Autodesk Fusion 360 part; units mm, degrees
(part 3 of 5)
  spline S763 degree 3 poles (27.3731, 3.8659) (27.3731, 3.7395) (27.3641, 3.6132) (27.346, 3.5681) knots 0 0 0 0 1 1 1 1
  spline S764 degree 3 poles (27.346, 3.5681) (27.337, 3.532) (26.967, 3.4959) (26.5157, 3.4868) knots 0 0 0 0 1 1 1 1
  spline S765 degree 3 poles (26.5157, 3.4868) (26.0645, 3.4778) (25.6222, 3.4598) (25.532, 3.4598) knots 0 0 0 0 1 1 1 1
  spline S766 degree 3 poles (25.532, 3.4598) (25.4327, 3.4507) (25.1981, 3.6132) (24.9995, 3.8208) knots 0 0 0 0 1 1 1 1
  spline S767 degree 3 poles (24.9995, 3.8208) (24.6566, 4.1727) (24.4851, 4.263) (24.4851, 4.1005) knots 0 0 0 0 1 1 1 1
  spline S768 degree 3 poles (24.4851, 4.1005) (24.4851, 4.0554) (24.5483, 3.9742) (24.6205, 3.911) knots 0 0 0 0 1 1 1 1
  spline S769 degree 3 poles (24.6205, 3.911) (24.9183, 3.6673) (24.7288, 3.4598) (24.2053, 3.4598) knots 0 0 0 0 1 1 1 1
  spline S770 degree 3 poles (24.2053, 3.4598) (23.9436, 3.4598) (23.9436, 3.4598) (24.088, 3.6854) knots 0 0 0 0 1 1 1 1
  spline S771 degree 3 poles (24.088, 3.6854) (24.1692, 3.8117) (24.2143, 3.9381) (24.1873, 3.9742) knots 0 0 0 0 1 1 1 1
  spline S772 degree 3 poles (24.1873, 3.9742) (24.097, 4.0554) (23.6728, 3.911) (23.6187, 3.7847) knots 0 0 0 0 1 1 1 1
  spline S773 degree 3 poles (23.6187, 3.7847) (23.5916, 3.7125) (23.4201, 3.4959) (23.2396, 3.2973) knots 0 0 0 0 1 1 1 1
  spline S774 degree 3 poles (23.2396, 3.2973) (22.9869, 3.0175) (22.8335, 2.9273) (22.6079, 2.9273) knots 0 0 0 0 1 1 1 1
  line L62 (22.6079, 2.9273) -> (22.3191, 2.9183)
  line L63 (22.3191, 2.9183) -> (22.3191, 3.4778)
  spline S775 degree 3 poles (19.9907, 3.3063) (20.2343, 3.3966) (20.2795, 3.3424) (20.1531, 3.0988) knots 0 0 0 0 1 1 1 1
  spline S776 degree 3 poles (20.1531, 3.0988) (20.0538, 2.9092) (20.0448, 2.9092) (19.9275, 3.0717) knots 0 0 0 0 1 1 1 1
  spline S777 degree 3 poles (19.9275, 3.0717) (19.8192, 3.2161) (19.8282, 3.2432) (19.9907, 3.3063) knots 0 0 0 0 1 1 1 1
  spline S778 degree 3 poles (19.4401, 3.0356) (19.386, 3.1078) (19.3679, 3.189) (19.404, 3.2161) knots 0 0 0 0 1 1 1 1
  spline S779 degree 3 poles (19.404, 3.2161) (19.4672, 3.2883) (19.7019, 3.1168) (19.7019, 2.9995) knots 0 0 0 0 1 1 1 1
  spline S780 degree 3 poles (19.7019, 2.9995) (19.7019, 2.8822) (19.5575, 2.9002) (19.4401, 3.0356) knots 0 0 0 0 1 1 1 1
  spline S781 degree 3 poles (20.83, 3.0988) (20.8029, 3.1439) (20.839, 3.189) (20.9112, 3.189) knots 0 0 0 0 1 1 1 1
  spline S782 degree 3 poles (20.9112, 3.189) (20.9924, 3.189) (21.0556, 3.1439) (21.0556, 3.0988) knots 0 0 0 0 1 1 1 1
  spline S783 degree 3 poles (21.0556, 3.0988) (21.0556, 3.0446) (21.0195, 3.0085) (20.9744, 3.0085) knots 0 0 0 0 1 1 1 1
  spline S784 degree 3 poles (20.9744, 3.0085) (20.9202, 3.0085) (20.857, 3.0446) (20.83, 3.0988) knots 0 0 0 0 1 1 1 1
  spline S785 degree 3 poles (17.8969, 3.2341) (18.1947, 3.4056) (18.3481, 3.3966) (18.1315, 3.2341) knots 0 0 0 0 1 1 1 1
  spline S786 degree 3 poles (18.1315, 3.2341) (18.0322, 3.1619) (17.8878, 3.0988) (17.8156, 3.0988) knots 0 0 0 0 1 1 1 1
  spline S787 degree 3 poles (17.8156, 3.0988) (17.7254, 3.1078) (17.7525, 3.1529) (17.8969, 3.2341) knots 0 0 0 0 1 1 1 1
  spline S788 degree 3 poles (20.9653, 3.3695) (20.9653, 3.4146) (20.9834, 3.4598) (21.0014, 3.4598) knots 0 0 0 0 1 1 1 1
  spline S789 degree 3 poles (21.0014, 3.4598) (21.0285, 3.4598) (21.0736, 3.4146) (21.1007, 3.3695) knots 0 0 0 0 1 1 1 1
  spline S790 degree 3 poles (21.1007, 3.3695) (21.1278, 3.3154) (21.1097, 3.2793) (21.0646, 3.2793) knots 0 0 0 0 1 1 1 1
  spline S791 degree 3 poles (21.0646, 3.2793) (21.0105, 3.2793) (20.9653, 3.3154) (20.9653, 3.3695) knots 0 0 0 0 1 1 1 1
  spline S792 degree 3 poles (-4.6205, 3.55) (-5.884, 3.7215) (-6.0645, 3.7576) (-6.1638, 3.8388) knots 0 0 0 0 1 1 1 1
  spline S793 degree 3 poles (-6.1638, 3.8388) (-6.2179, 3.8749) (-6.3262, 3.893) (-6.4075, 3.8569) knots 0 0 0 0 1 1 1 1
  spline S794 degree 3 poles (-6.4075, 3.8569) (-6.4797, 3.8298) (-6.6963, 3.8478) (-6.8768, 3.902) knots 0 0 0 0 1 1 1 1
  spline S795 degree 3 poles (-6.8768, 3.902) (-7.1475, 3.9742) (-7.2558, 3.9561) (-7.5356, 3.8027) knots 0 0 0 0 1 1 1 1
  spline S796 degree 3 poles (-7.5356, 3.8027) (-7.8334, 3.6403) (-7.9598, 3.6312) (-8.9976, 3.6764) knots 0 0 0 0 1 1 1 1
  spline S797 degree 3 poles (-8.9976, 3.6764) (-9.7828, 3.7215) (-10.3514, 3.7034) (-10.8929, 3.6132) knots 0 0 0 0 1 1 1 1
  spline S798 degree 3 poles (-10.8929, 3.6132) (-11.4976, 3.5139) (-11.8405, 3.5049) (-12.5535, 3.5861) knots 0 0 0 0 1 1 1 1
  spline S799 degree 3 poles (-12.5535, 3.5861) (-13.7719, 3.7215) (-13.5553, 3.8659) (-12.021, 3.9471) knots 0 0 0 0 1 1 1 1
  spline S800 degree 3 poles (-12.021, 3.9471) (-11.3802, 3.9832) (-10.586, 4.0374) (-10.2611, 4.0825) knots 0 0 0 0 1 1 1 1
  spline S801 degree 3 poles (-10.2611, 4.0825) (-9.9362, 4.1186) (-9.3947, 4.1186) (-9.0428, 4.0825) knots 0 0 0 0 1 1 1 1
  spline S802 degree 3 poles (-9.0428, 4.0825) (-8.6998, 4.0554) (-7.9237, 4.0644) (-7.328, 4.1096) knots 0 0 0 0 1 1 1 1
  spline S803 degree 3 poles (-7.328, 4.1096) (-6.5519, 4.1727) (-6.1548, 4.1727) (-5.9021, 4.0915) knots 0 0 0 0 1 1 1 1
  spline S804 degree 3 poles (-5.9021, 4.0915) (-5.3967, 3.9381) (-4.0519, 3.7305) (-3.5646, 3.7305) knots 0 0 0 0 1 1 1 1
  spline S805 degree 3 poles (-3.5646, 3.7305) (-3.3299, 3.7305) (-3.0321, 3.7756) (-2.8877, 3.8298) knots 0 0 0 0 1 1 1 1
  spline S806 degree 3 poles (-2.8877, 3.8298) (-2.5718, 3.9652) (3.7998, 4.0193) (3.872, 3.893) knots 0 0 0 0 1 1 1 1
  spline S807 degree 3 poles (3.872, 3.893) (3.8991, 3.8478) (3.9803, 3.8569) (4.0525, 3.92) knots 0 0 0 0 1 1 1 1
  spline S808 degree 3 poles (4.0525, 3.92) (4.224, 4.0644) (7.0849, 3.9471) (7.1752, 3.7937) knots 0 0 0 0 1 1 1 1
  spline S809 degree 3 poles (7.1752, 3.7937) (7.2203, 3.7125) (7.2654, 3.7125) (7.3466, 3.7937) knots 0 0 0 0 1 1 1 1
  spline S810 degree 3 poles (7.3466, 3.7937) (7.4279, 3.8749) (7.491, 3.8749) (7.5723, 3.8117) knots 0 0 0 0 1 1 1 1
  spline S811 degree 3 poles (7.5723, 3.8117) (7.6445, 3.7576) (7.7798, 3.7486) (7.8972, 3.7847) knots 0 0 0 0 1 1 1 1
  spline S812 degree 3 poles (7.8972, 3.7847) (8.1047, 3.8478) (8.574, 3.8749) (11.3989, 3.9381) knots 0 0 0 0 1 1 1 1
  spline S813 degree 3 poles (11.3989, 3.9381) (13.0865, 3.9832) (13.4746, 3.9471) (13.4746, 3.7666) knots 0 0 0 0 1 1 1 1
  spline S814 degree 3 poles (13.4746, 3.7666) (13.4746, 3.6673) (13.1317, 3.6403) (11.5974, 3.6222) knots 0 0 0 0 1 1 1 1
  spline S815 degree 3 poles (11.5974, 3.6222) (8.2762, 3.5861) (4.242, 3.6312) (4.1879, 3.7125) knots 0 0 0 0 1 1 1 1
  spline S816 degree 3 poles (4.1879, 3.7125) (4.1067, 3.8208) (3.4569, 3.8388) (3.4569, 3.7305) knots 0 0 0 0 1 1 1 1
  spline S817 degree 3 poles (3.4569, 3.7305) (3.4569, 3.6764) (3.0056, 3.6583) (2.1212, 3.6854) knots 0 0 0 0 1 1 1 1
  spline S818 degree 3 poles (2.1212, 3.6854) (-0.2975, 3.7756) (-0.6405, 3.7666) (-1.7325, 3.6132) knots 0 0 0 0 1 1 1 1
  spline S819 degree 3 poles (-1.7325, 3.6132) (-3.5556, 3.3605) (-3.3209, 3.3695) (-4.6205, 3.55) knots 0 0 0 0 1 1 1 1
  spline S820 degree 3 poles (20.7397, 3.6403) (20.7126, 3.6854) (20.7668, 3.7305) (20.8661, 3.7305) knots 0 0 0 0 1 1 1 1
  spline S821 degree 3 poles (20.8661, 3.7305) (20.9653, 3.7305) (21.0736, 3.6854) (21.1007, 3.6403) knots 0 0 0 0 1 1 1 1
  spline S822 degree 3 poles (21.1007, 3.6403) (21.1278, 3.5861) (21.0736, 3.55) (20.9744, 3.55) knots 0 0 0 0 1 1 1 1
  spline S823 degree 3 poles (20.9744, 3.55) (20.8751, 3.55) (20.7668, 3.5861) (20.7397, 3.6403) knots 0 0 0 0 1 1 1 1
  spline S824 degree 3 poles (18.0142, 3.6042) (18.0413, 3.6312) (18.1225, 3.6403) (18.1857, 3.6132) knots 0 0 0 0 1 1 1 1
  spline S825 degree 3 poles (18.1857, 3.6132) (18.2579, 3.5861) (18.2308, 3.559) (18.1315, 3.559) knots 0 0 0 0 1 1 1 1
  spline S826 degree 3 poles (18.1315, 3.559) (18.0322, 3.55) (17.9781, 3.5771) (18.0142, 3.6042) knots 0 0 0 0 1 1 1 1
  spline S827 degree 3 poles (-26.7769, 3.6403) (-26.7769, 3.6854) (-26.7408, 3.7305) (-26.6866, 3.7305) knots 0 0 0 0 1 1 1 1
  spline S828 degree 3 poles (-26.6866, 3.7305) (-26.6415, 3.7305) (-26.5964, 3.6854) (-26.5964, 3.6403) knots 0 0 0 0 1 1 1 1
  spline S829 degree 3 poles (-26.5964, 3.6403) (-26.5964, 3.5861) (-26.6415, 3.55) (-26.6866, 3.55) knots 0 0 0 0 1 1 1 1
  spline S830 degree 3 poles (-26.6866, 3.55) (-26.7408, 3.55) (-26.7769, 3.5861) (-26.7769, 3.6403) knots 0 0 0 0 1 1 1 1
  spline S831 degree 3 poles (-30.0891, 3.7486) (-30.062, 3.8208) (-30.0349, 3.7937) (-30.0349, 3.6944) knots 0 0 0 0 1 1 1 1
  spline S832 degree 3 poles (-30.0349, 3.6944) (-30.0259, 3.5951) (-30.053, 3.541) (-30.08, 3.5771) knots 0 0 0 0 1 1 1 1
  spline S833 degree 3 poles (-30.08, 3.5771) (-30.1071, 3.6042) (-30.1161, 3.6854) (-30.0891, 3.7486) knots 0 0 0 0 1 1 1 1
  spline S834 degree 3 poles (-31.4428, 3.8388) (-31.4157, 3.902) (-31.3977, 3.8569) (-31.3977, 3.7305) knots 0 0 0 0 1 1 1 1
  spline S835 degree 3 poles (-31.3977, 3.7305) (-31.3977, 3.6042) (-31.4157, 3.559) (-31.4428, 3.6132) knots 0 0 0 0 1 1 1 1
  spline S836 degree 3 poles (-31.4428, 3.6132) (-31.4609, 3.6764) (-31.4609, 3.7847) (-31.4428, 3.8388) knots 0 0 0 0 1 1 1 1
  spline S837 degree 3 poles (19.7289, 3.7847) (19.756, 3.8117) (19.8372, 3.8208) (19.9004, 3.7937) knots 0 0 0 0 1 1 1 1
  spline S838 degree 3 poles (19.9004, 3.7937) (19.9726, 3.7666) (19.9455, 3.7395) (19.8463, 3.7395) knots 0 0 0 0 1 1 1 1
  spline S839 degree 3 poles (19.8463, 3.7395) (19.747, 3.7305) (19.6928, 3.7576) (19.7289, 3.7847) knots 0 0 0 0 1 1 1 1
  spline S840 degree 3 poles (20.7397, 3.911) (20.7126, 3.9561) (20.7668, 4.0013) (20.8661, 4.0013) knots 0 0 0 0 1 1 1 1
  spline S841 degree 3 poles (20.8661, 4.0013) (20.9744, 4.0013) (21.0556, 3.9561) (21.0556, 3.911) knots 0 0 0 0 1 1 1 1
  spline S842 degree 3 poles (21.0556, 3.911) (21.0556, 3.8569) (21.0014, 3.8208) (20.9292, 3.8208) knots 0 0 0 0 1 1 1 1
  spline S843 degree 3 poles (20.9292, 3.8208) (20.857, 3.8208) (20.7668, 3.8569) (20.7397, 3.911) knots 0 0 0 0 1 1 1 1
  spline S844 degree 3 poles (19.8824, 4.0915) (19.8824, 4.2359) (20.0809, 4.2991) (20.1621, 4.1727) knots 0 0 0 0 1 1 1 1
  spline S845 degree 3 poles (20.1621, 4.1727) (20.3065, 3.9381) (20.2614, 3.8027) (20.0629, 3.911) knots 0 0 0 0 1 1 1 1
  spline S846 degree 3 poles (20.0629, 3.911) (19.9636, 3.9652) (19.8824, 4.0464) (19.8824, 4.0915) knots 0 0 0 0 1 1 1 1
  spline S847 degree 3 poles (18.0413, 3.8749) (17.96, 3.902) (17.9149, 3.9652) (17.942, 4.0103) knots 0 0 0 0 1 1 1 1
  spline S848 degree 3 poles (17.942, 4.0103) (18.0052, 4.1005) (18.2579, 4.0103) (18.2579, 3.902) knots 0 0 0 0 1 1 1 1
  spline S849 degree 3 poles (18.2579, 3.902) (18.2579, 3.8027) (18.2308, 3.8027) (18.0413, 3.8749) knots 0 0 0 0 1 1 1 1
  spline S850 degree 3 poles (-26.1451, 4.0103) (-26.1451, 4.0644) (-26.109, 4.0735) (-26.0549, 4.0464) knots 0 0 0 0 1 1 1 1
  spline S851 degree 3 poles (-26.0549, 4.0464) (-26.0098, 4.0193) (-25.9646, 3.9471) (-25.9646, 3.902) knots 0 0 0 0 1 1 1 1
  spline S852 degree 3 poles (-25.9646, 3.902) (-25.9646, 3.8478) (-26.0098, 3.8388) (-26.0549, 3.8659) knots 0 0 0 0 1 1 1 1
  spline S853 degree 3 poles (-26.0549, 3.8659) (-26.109, 3.893) (-26.1451, 3.9652) (-26.1451, 4.0103) knots 0 0 0 0 1 1 1 1
  spline S854 degree 3 poles (-26.9574, 3.902) (-26.9574, 3.9381) (-26.8762, 4.0825) (-26.7679, 4.2179) knots 0 0 0 0 1 1 1 1
  spline S855 degree 3 poles (-26.7679, 4.2179) (-26.5513, 4.4976) (-26.2264, 4.5428) (-26.2986, 4.281) knots 0 0 0 0 1 1 1 1
  spline S856 degree 3 poles (-26.2986, 4.281) (-26.3256, 4.1637) (-26.3978, 4.1276) (-26.5242, 4.1637) knots 0 0 0 0 1 1 1 1
  spline S857 degree 3 poles (-26.5242, 4.1637) (-26.6866, 4.1998) (-26.7047, 4.1818) (-26.6686, 4.0193) knots 0 0 0 0 1 1 1 1
  spline S858 degree 3 poles (-26.6686, 4.0193) (-26.6235, 3.8659) (-26.6505, 3.8208) (-26.7859, 3.8208) knots 0 0 0 0 1 1 1 1
  spline S859 degree 3 poles (-26.7859, 3.8208) (-26.8762, 3.8208) (-26.9574, 3.8569) (-26.9574, 3.902) knots 0 0 0 0 1 1 1 1
  spline S860 degree 3 poles (19.395, 3.9922) (19.3679, 4.0374) (19.404, 4.1005) (19.4853, 4.1276) knots 0 0 0 0 1 1 1 1
  spline S861 degree 3 poles (19.4853, 4.1276) (19.6658, 4.1998) (19.747, 4.1366) (19.6567, 4.0103) knots 0 0 0 0 1 1 1 1
  spline S862 degree 3 poles (19.6567, 4.0103) (19.5845, 3.893) (19.4582, 3.8839) (19.395, 3.9922) knots 0 0 0 0 1 1 1 1
  spline S863 degree 3 poles (-25.7841, 3.9471) (-25.7841, 3.9742) (-25.748, 4.0193) (-25.6939, 4.0464) knots 0 0 0 0 1 1 1 1
  spline S864 degree 3 poles (-25.6939, 4.0464) (-25.6488, 4.0735) (-25.6036, 4.0554) (-25.6036, 4.0103) knots 0 0 0 0 1 1 1 1
  spline S865 degree 3 poles (-25.6036, 4.0103) (-25.6036, 3.9561) (-25.6488, 3.911) (-25.6939, 3.911) knots 0 0 0 0 1 1 1 1
  spline S866 degree 3 poles (-25.6939, 3.911) (-25.748, 3.911) (-25.7841, 3.9291) (-25.7841, 3.9471) knots 0 0 0 0 1 1 1 1
  spline S867 degree 3 poles (-26.0368, 4.272) (-26.1451, 4.4525) (-26.091, 4.4976) (-25.8383, 4.3984) knots 0 0 0 0 1 1 1 1
  spline S868 degree 3 poles (-25.8383, 4.3984) (-25.7661, 4.3713) (-25.73, 4.2901) (-25.7571, 4.2179) knots 0 0 0 0 1 1 1 1
  spline S869 degree 3 poles (-25.7571, 4.2179) (-25.8202, 4.0464) (-25.9015, 4.0554) (-26.0368, 4.272) knots 0 0 0 0 1 1 1 1
  spline S870 degree 3 poles (19.2506, 4.4074) (19.3138, 4.4886) (19.386, 4.5247) (19.4131, 4.4976) knots 0 0 0 0 1 1 1 1
  spline S871 degree 3 poles (19.4131, 4.4976) (19.4401, 4.4796) (19.404, 4.3984) (19.3409, 4.3171) knots 0 0 0 0 1 1 1 1
  spline S872 degree 3 poles (19.3409, 4.3171) (19.2777, 4.2359) (19.2055, 4.1998) (19.1784, 4.2269) knots 0 0 0 0 1 1 1 1
  spline S873 degree 3 poles (19.1784, 4.2269) (19.1513, 4.2449) (19.1874, 4.3262) (19.2506, 4.4074) knots 0 0 0 0 1 1 1 1
  spline S874 degree 3 poles (19.5845, 4.5337) (19.5575, 4.6601) (19.5845, 4.6872) (19.7109, 4.6601) knots 0 0 0 0 1 1 1 1
  spline S875 degree 3 poles (19.7109, 4.6601) (19.9094, 4.6059) (19.9365, 4.4886) (19.765, 4.4254) knots 0 0 0 0 1 1 1 1
  spline S876 degree 2 poles (19.765, 4.4254) (19.7109, 4.3984) (19.6477, 4.3713) knots 0 0 0 1 1 1
  spline S877 degree 3 poles (19.6477, 4.3713) (19.6387, 4.3623) (19.6116, 4.4345) (19.5845, 4.5337) knots 0 0 0 0 1 1 1 1
  spline S878 degree 3 poles (19.1152, 4.7233) (19.0882, 4.7684) (19.1423, 4.8135) (19.2506, 4.8135) knots 0 0 0 0 1 1 1 1
  spline S879 degree 3 poles (19.2506, 4.8135) (19.3589, 4.8135) (19.4131, 4.7684) (19.386, 4.7233) knots 0 0 0 0 1 1 1 1
  spline S880 degree 3 poles (19.386, 4.7233) (19.3589, 4.6691) (19.2957, 4.633) (19.2506, 4.633) knots 0 0 0 0 1 1 1 1
  spline S881 degree 3 poles (19.2506, 4.633) (19.2055, 4.633) (19.1423, 4.6691) (19.1152, 4.7233) knots 0 0 0 0 1 1 1 1
  spline S882 degree 3 poles (18.664, 4.8135) (18.6369, 4.8586) (18.6459, 4.9038) (18.7001, 4.9038) knots 0 0 0 0 1 1 1 1
  spline S883 degree 3 poles (18.7001, 4.9038) (18.7452, 4.9038) (18.8174, 4.8586) (18.8445, 4.8135) knots 0 0 0 0 1 1 1 1
  spline S884 degree 3 poles (18.8445, 4.8135) (18.8716, 4.7594) (18.8625, 4.7233) (18.8084, 4.7233) knots 0 0 0 0 1 1 1 1
  spline S885 degree 3 poles (18.8084, 4.7233) (18.7633, 4.7233) (18.6911, 4.7594) (18.664, 4.8135) knots 0 0 0 0 1 1 1 1
  spline S886 degree 3 poles (-25.5766, 5.1926) (-25.5495, 5.2557) (-25.5314, 5.2106) (-25.5314, 5.0843) knots 0 0 0 0 1 1 1 1
  spline S887 degree 3 poles (-25.5314, 5.0843) (-25.5314, 4.9579) (-25.5495, 4.9128) (-25.5766, 4.9669) knots 0 0 0 0 1 1 1 1
  spline S888 degree 3 poles (-25.5766, 4.9669) (-25.5946, 5.0301) (-25.5946, 5.1384) (-25.5766, 5.1926) knots 0 0 0 0 1 1 1 1
  spline S889 degree 3 poles (1.5616, -7.1897) (1.5616, -7.1446) (1.4984, -7.0995) (1.4262, -7.0995) knots 0 0 0 0 1 1 1 1
  spline S890 degree 3 poles (1.4262, -7.0995) (1.354, -7.0995) (1.2909, -7.1446) (1.2909, -7.1897) knots 0 0 0 0 1 1 1 1
  spline S891 degree 3 poles (1.2909, -7.1897) (1.2909, -7.2439) (1.354, -7.28) (1.4262, -7.28) knots 0 0 0 0 1 1 1 1
  spline S892 degree 3 poles (1.4262, -7.28) (1.4984, -7.28) (1.5616, -7.2439) (1.5616, -7.1897) knots 0 0 0 0 1 1 1 1
  spline S893 degree 3 poles (-0.2885, -7.0995) (-0.2614, -7.0544) (-0.2795, -7.0092) (-0.3246, -7.0092) knots 0 0 0 0 1 1 1 1
  spline S894 degree 3 poles (-0.3246, -7.0092) (-0.3788, -7.0092) (-0.4239, -7.0544) (-0.4239, -7.0995) knots 0 0 0 0 1 1 1 1
  spline S895 degree 3 poles (-0.4239, -7.0995) (-0.4239, -7.1536) (-0.4058, -7.1897) (-0.3878, -7.1897) knots 0 0 0 0 1 1 1 1
  spline S896 degree 3 poles (-0.3878, -7.1897) (-0.3607, -7.1897) (-0.3156, -7.1536) (-0.2885, -7.0995) knots 0 0 0 0 1 1 1 1
  spline S897 degree 3 poles (15.406, -6.91) (15.5323, -6.8107) (15.6406, -6.6573) (15.6406, -6.576) knots 0 0 0 0 1 1 1 1
  spline S898 degree 3 poles (15.6406, -6.576) (15.6406, -6.4858) (15.6135, -6.4587) (15.5684, -6.5129) knots 0 0 0 0 1 1 1 1
  spline S899 degree 3 poles (15.5684, -6.5129) (15.4872, -6.6302) (15.1894, -6.8197) (14.9818, -6.8829) knots 0 0 0 0 1 1 1 1
  spline S900 degree 3 poles (14.9818, -6.8829) (14.9006, -6.919) (14.8284, -6.9731) (14.8284, -7.0183) knots 0 0 0 0 1 1 1 1
  spline S901 degree 3 poles (14.8284, -7.0183) (14.8284, -7.1627) (15.1623, -7.0995) (15.406, -6.91) knots 0 0 0 0 1 1 1 1
  spline S902 degree 3 poles (-1.3715, -7.0092) (-1.3354, -6.9461) (-1.1549, -6.937) (-0.9112, -6.9731) knots 0 0 0 0 1 1 1 1
  spline S903 degree 3 poles (-0.9112, -6.9731) (-0.6224, -7.0092) (-0.5141, -7.0002) (-0.5141, -6.919) knots 0 0 0 0 1 1 1 1
  spline S904 degree 3 poles (-0.5141, -6.919) (-0.5141, -6.8378) (-0.4058, -6.8197) (-0.1351, -6.8558) knots 0 0 0 0 1 1 1 1
  spline S905 degree 3 poles (-0.1351, -6.8558) (0.3162, -6.919) (1.1555, -6.7204) (1.4714, -6.4768) knots 0 0 0 0 1 1 1 1
  spline S906 degree 3 poles (1.4714, -6.4768) (1.6699, -6.3324) (1.697, -6.2421) (1.6789, -5.827) knots 0 0 0 0 1 1 1 1
  spline S907 degree 3 poles (1.6789, -5.827) (1.6699, -5.5562) (1.6067, -5.0598) (1.5345, -4.7079) knots 0 0 0 0 1 1 1 1
  spline S908 degree 3 poles (1.5345, -4.7079) (1.4353, -4.2476) (1.4262, -4.04) (1.4984, -3.9227) knots 0 0 0 0 1 1 1 1
  spline S909 degree 3 poles (1.4984, -3.9227) (1.6067, -3.7602) (1.6067, -3.7512) (0.8216, -2.9751) knots 0 0 0 0 1 1 1 1
  spline S910 degree 3 poles (0.8216, -2.9751) (0.4876, -2.6502) (0.4154, -2.6141) (0.2169, -2.6863) knots 0 0 0 0 1 1 1 1
  spline S911 degree 3 poles (0.2169, -2.6863) (-0.0719, -2.8036) (-1.0737, -2.939) (-2.0033, -2.9931) knots 0 0 0 0 1 1 1 1
  spline S912 degree 3 poles (-2.0033, -2.9931) (-3.1585, -3.0653) (-3.4834, -3.1195) (-3.8173, -3.2729) knots 0 0 0 0 1 1 1 1
  spline S913 degree 3 poles (-3.8173, -3.2729) (-4.2144, -3.4624) (-4.3407, -3.6971) (-4.3137, -4.2025) knots 0 0 0 0 1 1 1 1
  spline S914 degree 3 poles (-4.3137, -4.2025) (-4.3046, -4.4461) (-4.3498, -4.6357) (-4.4129, -4.6718) knots 0 0 0 0 1 1 1 1
  spline S915 degree 3 poles (-4.4129, -4.6718) (-4.5032, -4.7259) (-4.4851, -4.7801) (-4.3588, -4.8703) knots 0 0 0 0 1 1 1 1
  spline S916 degree 3 poles (-4.3588, -4.8703) (-4.2595, -4.9425) (-4.2234, -5.0237) (-4.2776, -5.0508) knots 0 0 0 0 1 1 1 1
  spline S917 degree 3 poles (-4.2776, -5.0508) (-4.422, -5.1411) (-4.2595, -5.845) (-4.0519, -6.0075) knots 0 0 0 0 1 1 1 1
  spline S918 degree 3 poles (-4.0519, -6.0075) (-3.9527, -6.0887) (-3.8444, -6.2421) (-3.8083, -6.3594) knots 0 0 0 0 1 1 1 1
  spline S919 degree 3 poles (-3.8083, -6.3594) (-3.7722, -6.4677) (-3.6007, -6.6663) (-3.4202, -6.7836) knots 0 0 0 0 1 1 1 1
  spline S920 degree 3 poles (-3.4202, -6.7836) (-3.0772, -7.0092) (-2.6982, -7.0544) (-1.9852, -6.9551) knots 0 0 0 0 1 1 1 1
  spline S921 degree 3 poles (-1.9852, -6.9551) (-1.7325, -6.919) (-1.5971, -6.937) (-1.5971, -7.0002) knots 0 0 0 0 1 1 1 1
  spline S922 degree 3 poles (-1.5971, -7.0002) (-1.5971, -7.1266) (-1.4437, -7.1266) (-1.3715, -7.0092) knots 0 0 0 0 1 1 1 1
  spline S923 degree 3 poles (-2.987, -6.2511) (-2.8155, -5.7006) (-2.7975, -5.6826) (-2.2108, -5.5562) knots 0 0 0 0 1 1 1 1
  spline S924 degree 3 poles (-2.2108, -5.5562) (-1.7145, -5.4479) (-1.6784, -5.4299) (-1.9491, -5.4028) knots 0 0 0 0 1 1 1 1
  spline S925 degree 3 poles (-1.9491, -5.4028) (-2.2289, -5.3757) (-2.2469, -5.3577) (-2.1928, -5.105) knots 0 0 0 0 1 1 1 1
  spline S926 degree 3 poles (-2.1928, -5.105) (-2.1296, -4.762) (-2.2108, -4.771) (-2.3282, -5.114) knots 0 0 0 0 1 1 1 1
  spline S927 degree 3 poles (-2.3282, -5.114) (-2.4996, -5.6013) (-2.8606, -5.3577) (-2.8606, -4.762) knots 0 0 0 0 1 1 1 1
  spline S928 degree 3 poles (-2.8606, -4.762) (-2.8606, -4.6086) (-2.9058, -4.4822) (-2.9509, -4.4822) knots 0 0 0 0 1 1 1 1
  spline S929 degree 3 poles (-2.9509, -4.4822) (-3.005, -4.4822) (-3.0411, -4.5454) (-3.0411, -4.6357) knots 0 0 0 0 1 1 1 1
  spline S930 degree 3 poles (-3.0411, -4.6357) (-3.0411, -4.762) (-3.0592, -4.762) (-3.2216, -4.6176) knots 0 0 0 0 1 1 1 1
  spline S931 degree 3 poles (-3.2216, -4.6176) (-3.5195, -4.3559) (-3.5104, -4.5093) (-3.2126, -4.8703) knots 0 0 0 0 1 1 1 1
  spline S932 degree 3 poles (-3.2126, -4.8703) (-2.9148, -5.2313) (-2.8697, -5.5291) (-3.0321, -6.0436) knots 0 0 0 0 1 1 1 1
  spline S933 degree 3 poles (-3.0321, -6.0436) (-3.2397, -6.6663) (-3.4021, -6.4587) (-3.727, -5.1862) knots 0 0 0 0 1 1 1 1
  spline S934 degree 3 poles (-3.727, -5.1862) (-3.8714, -4.5996) (-3.9436, -4.1212) (-3.9075, -3.9859) knots 0 0 0 0 1 1 1 1
  spline S935 degree 3 poles (-3.9075, -3.9859) (-3.8353, -3.688) (-3.3841, -3.4895) (-2.7884, -3.4895) knots 0 0 0 0 1 1 1 1
  spline S936 degree 3 poles (-2.7884, -3.4895) (-2.3011, -3.4895) (-2.256, -3.5436) (-2.0574, -4.2837) knots 0 0 0 0 1 1 1 1
  spline S937 degree 3 poles (-2.0574, -4.2837) (-1.9491, -4.6627) (-1.6423, -5.114) (-1.4888, -5.114) knots 0 0 0 0 1 1 1 1
  spline S938 degree 3 poles (-1.4888, -5.114) (-1.4347, -5.114) (-1.4618, -5.0328) (-1.552, -4.9335) knots 0 0 0 0 1 1 1 1
  spline S939 degree 3 poles (-1.552, -4.9335) (-1.7776, -4.6898) (-1.6874, -4.6357) (-1.0286, -4.5905) knots 0 0 0 0 1 1 1 1
  spline S940 degree 3 poles (-1.0286, -4.5905) (-0.5051, -4.5544) (-0.46, -4.5725) (-0.3427, -4.7801) knots 0 0 0 0 1 1 1 1
  spline S941 degree 3 poles (-0.3427, -4.7801) (-0.1802, -5.0779) (-0.2795, -5.2042) (-0.6315, -5.1501) knots 0 0 0 0 1 1 1 1
  spline S942 degree 3 poles (-0.6315, -5.1501) (-0.9112, -5.114) (-0.9112, -5.114) (-0.6946, -5.2223) knots 0 0 0 0 1 1 1 1
  spline S943 degree 3 poles (-0.6946, -5.2223) (-0.5683, -5.2764) (-0.451, -5.3396) (-0.4329, -5.3577) knots 0 0 0 0 1 1 1 1
  spline S944 degree 3 poles (-0.4329, -5.3577) (-0.4149, -5.3757) (-0.469, -5.466) (-0.5593, -5.5652) knots 0 0 0 0 1 1 1 1
  spline S945 degree 3 poles (-0.5593, -5.5652) (-0.6495, -5.6645) (-0.6766, -5.7457) (-0.6224, -5.7457) knots 0 0 0 0 1 1 1 1
  spline S946 degree 3 poles (-0.6224, -5.7457) (-0.5683, -5.7457) (-0.4329, -5.6104) (-0.3246, -5.4569) knots 0 0 0 0 1 1 1 1
  spline S947 degree 3 poles (-0.3246, -5.4569) (-0.2163, -5.2945) (-0.108, -5.1411) (-0.099, -5.123) knots 0 0 0 0 1 1 1 1
  spline S948 degree 3 poles (-0.099, -5.123) (-0.0809, -5.105) (0.0635, -5.2403) (0.2349, -5.4208) knots 0 0 0 0 1 1 1 1
  spline S949 degree 3 poles (0.2349, -5.4208) (0.4064, -5.6013) (0.623, -5.7457) (0.7133, -5.7457) knots 0 0 0 0 1 1 1 1
  spline S950 degree 3 poles (0.7133, -5.7457) (0.8757, -5.7367) (0.8757, -5.7367) (0.7133, -5.6104) knots 0 0 0 0 1 1 1 1
  spline S951 degree 3 poles (0.7133, -5.6104) (0.5418, -5.484) (0.5508, -5.475) (0.7584, -5.3938) knots 0 0 0 0 1 1 1 1
  spline S952 degree 3 poles (0.7584, -5.3938) (0.9569, -5.3125) (0.9479, -5.3035) (0.6411, -5.3035) knots 0 0 0 0 1 1 1 1
  spline S953 degree 3 poles (0.6411, -5.3035) (0.3793, -5.2945) (0.271, -5.2403) (0.1537, -5.0689) knots 0 0 0 0 1 1 1 1
  spline S954 degree 3 poles (0.1537, -5.0689) (-0.0178, -4.7981) (0.0183, -4.744) (0.4606, -4.6086) knots 0 0 0 0 1 1 1 1
  spline S955 degree 3 poles (0.4606, -4.6086) (0.8577, -4.4822) (0.5689, -4.4461) (0.1537, -4.5635) knots 0 0 0 0 1 1 1 1
  spline S956 degree 3 poles (0.1537, -4.5635) (-0.0268, -4.6176) (-0.1802, -4.6086) (-0.2975, -4.5364) knots 0 0 0 0 1 1 1 1
  spline S957 degree 3 poles (-0.2975, -4.5364) (-0.3878, -4.4822) (-0.7759, -4.4371) (-1.1459, -4.4371) knots 0 0 0 0 1 1 1 1
  line L64 (-1.1459, -4.4371) -> (-1.8137, -4.4371)
  line L65 (-1.8137, -4.4371) -> (-1.9762, -4.0039)
  spline S958 degree 3 poles (-1.9762, -4.0039) (-2.1025, -3.679) (-2.1116, -3.5617) (-2.0213, -3.5346) knots 0 0 0 0 1 1 1 1
  spline S959 degree 3 poles (-2.0213, -3.5346) (-1.9672, -3.5075) (-1.3715, -3.5256) (-0.7037, -3.5707) knots 0 0 0 0 1 1 1 1
  spline S960 degree 3 poles (-0.7037, -3.5707) (0.4154, -3.6429) (0.5147, -3.661) (0.7313, -3.8776) knots 0 0 0 0 1 1 1 1
  spline S961 degree 3 poles (0.7313, -3.8776) (0.9208, -4.0671) (0.984, -4.2656) (1.0743, -4.8432) knots 0 0 0 0 1 1 1 1
  spline S962 degree 3 poles (1.0743, -4.8432) (1.1916, -5.6826) (1.1555, -5.9894) (0.9299, -6.1067) knots 0 0 0 0 1 1 1 1
  spline S963 degree 3 poles (0.9299, -6.1067) (0.8396, -6.1609) (0.244, -6.2421) (-0.3968, -6.2963) knots 0 0 0 0 1 1 1 1
  spline S964 degree 3 poles (-0.3968, -6.2963) (-1.0286, -6.3504) (-1.8408, -6.4226) (-2.1838, -6.4587) knots 0 0 0 0 1 1 1 1
  spline S965 degree 3 poles (-2.1838, -6.4587) (-2.9509, -6.5399) (-3.0682, -6.5038) (-2.987, -6.2511) knots 0 0 0 0 1 1 1 1
  spline S966 degree 3 poles (0.2079, -3.3992) (0.2079, -3.3541) (0.253, -3.309) (0.3071, -3.309) knots 0 0 0 0 1 1 1 1
  spline S967 degree 3 poles (0.3071, -3.309) (0.3523, -3.309) (0.3703, -3.3541) (0.3432, -3.3992) knots 0 0 0 0 1 1 1 1
  spline S968 degree 3 poles (0.3432, -3.3992) (0.3162, -3.4534) (0.271, -3.4895) (0.244, -3.4895) knots 0 0 0 0 1 1 1 1
  spline S969 degree 3 poles (0.244, -3.4895) (0.2259, -3.4895) (0.2079, -3.4534) (0.2079, -3.3992) knots 0 0 0 0 1 1 1 1
  spline S970 degree 3 poles (4.3594, -6.919) (4.3594, -6.8739) (4.3142, -6.8287) (4.2691, -6.8287) knots 0 0 0 0 1 1 1 1
  spline S971 degree 3 poles (4.2691, -6.8287) (4.215, -6.8287) (4.1789, -6.8739) (4.1789, -6.919) knots 0 0 0 0 1 1 1 1
  spline S972 degree 3 poles (4.1789, -6.919) (4.1789, -6.9731) (4.215, -7.0092) (4.2691, -7.0092) knots 0 0 0 0 1 1 1 1
  spline S973 degree 3 poles (4.2691, -7.0092) (4.3142, -7.0092) (4.3594, -6.9731) (4.3594, -6.919) knots 0 0 0 0 1 1 1 1
  spline S974 degree 3 poles (4.5399, -6.6031) (4.8287, -6.5309) (5.0723, -6.5129) (5.1175, -6.558) knots 0 0 0 0 1 1 1 1
  spline S975 degree 3 poles (5.1175, -6.558) (5.1626, -6.6031) (5.2709, -6.6031) (5.3702, -6.549) knots 0 0 0 0 1 1 1 1
  spline S976 degree 3 poles (5.3702, -6.549) (5.4965, -6.4858) (5.5777, -6.4858) (5.668, -6.558) knots 0 0 0 0 1 1 1 1
  spline S977 degree 3 poles (5.668, -6.558) (5.7582, -6.6302) (5.8395, -6.6302) (5.9748, -6.567) knots 0 0 0 0 1 1 1 1
  spline S978 degree 3 poles (5.9748, -6.567) (6.0741, -6.5129) (6.2275, -6.4677) (6.3268, -6.4677) knots 0 0 0 0 1 1 1 1
  spline S979 degree 3 poles (6.3268, -6.4677) (6.4261, -6.4677) (6.5524, -6.4046) (6.6156, -6.3324) knots 0 0 0 0 1 1 1 1
  spline S980 degree 3 poles (6.6156, -6.3324) (6.7059, -6.2241) (6.9044, -6.197) (7.473, -6.206) knots 0 0 0 0 1 1 1 1
  spline S981 degree 3 poles (7.473, -6.206) (8.8358, -6.2421) (9.1607, -5.7999) (8.7906, -4.4281) knots 0 0 0 0 1 1 1 1
  spline S982 degree 3 poles (8.7906, -4.4281) (8.2852, -2.5148) (8.3033, -2.5509) (7.6986, -2.6321) knots 0 0 0 0 1 1 1 1
  spline S983 degree 3 poles (7.6986, -2.6321) (7.3647, -2.6772) (7.2022, -2.6502) (6.8232, -2.4516) knots 0 0 0 0 1 1 1 1
  spline S984 degree 3 poles (6.8232, -2.4516) (6.4712, -2.2801) (6.3088, -2.244) (6.1914, -2.3072) knots 0 0 0 0 1 1 1 1
  spline S985 degree 3 poles (6.1914, -2.3072) (5.9478, -2.4336) (5.6951, -2.5238) (5.4875, -2.5509) knots 0 0 0 0 1 1 1 1
  spline S986 degree 3 poles (5.4875, -2.5509) (4.7745, -2.6411) (4.4947, -2.6682) (3.7727, -2.7224) knots 0 0 0 0 1 1 1 1
  spline S987 degree 3 poles (3.7727, -2.7224) (2.78, -2.8036) (2.3197, -2.9751) (2.1392, -3.318) knots 0 0 0 0 1 1 1 1
  spline S988 degree 3 poles (2.1392, -3.318) (2.0219, -3.5527) (2.0219, -3.679) (2.1573, -4.5003) knots 0 0 0 0 1 1 1 1
  spline S989 degree 3 poles (2.1573, -4.5003) (2.3197, -5.5652) (2.5634, -6.215) (2.8522, -6.3685) knots 0 0 0 0 1 1 1 1
  spline S990 degree 3 poles (2.8522, -6.3685) (3.0507, -6.4677) (3.9171, -6.7385) (3.9984, -6.7295) knots 0 0 0 0 1 1 1 1
  spline S991 degree 3 poles (3.9984, -6.7295) (4.0254, -6.7295) (4.2691, -6.6663) (4.5399, -6.6031) knots 0 0 0 0 1 1 1 1
  spline S992 degree 3 poles (3.0959, -6.0345) (2.9605, -5.9262) (2.8341, -5.6104) (2.6807, -5.0328) knots 0 0 0 0 1 1 1 1
  spline S993 degree 3 poles (2.6807, -5.0328) (2.419, -4.031) (2.41, -3.661) (2.6175, -3.4714) knots 0 0 0 0 1 1 1 1
  spline S994 degree 3 poles (2.6175, -3.4714) (2.8522, -3.2639) (3.0417, -3.2278) (4.0435, -3.2007) knots 0 0 0 0 1 1 1 1
  line L66 (4.0435, -3.2007) -> (4.946, -3.1826)
  line L67 (4.946, -3.1826) -> (5.0272, -3.6429)
  spline S995 degree 3 poles (5.0272, -3.6429) (5.0994, -4.0942) (5.0994, -4.1212) (4.7655, -4.5274) knots 0 0 0 0 1 1 1 1
  spline S996 degree 3 poles (4.7655, -4.5274) (4.576, -4.753) (4.4496, -4.9696) (4.4857, -5.0057) knots 0 0 0 0 1 1 1 1
  spline S997 degree 3 poles (4.4857, -5.0057) (4.5218, -5.0418) (4.6301, -4.9696) (4.7204, -4.8432) knots 0 0 0 0 1 1 1 1
  spline S998 degree 3 poles (4.7204, -4.8432) (4.8557, -4.6627) (4.9099, -4.6357) (5.0001, -4.7349) knots 0 0 0 0 1 1 1 1
  spline S999 degree 3 poles (5.0001, -4.7349) (5.1806, -4.9064) (5.2799, -4.8613) (5.1716, -4.6627) knots 0 0 0 0 1 1 1 1
  spline S1000 degree 3 poles (5.1716, -4.6627) (5.0994, -4.5183) (5.0994, -4.41) (5.1897, -4.2115) knots 0 0 0 0 1 1 1 1
  spline S1001 degree 3 poles (5.1897, -4.2115) (5.3341, -3.8776) (5.6048, -3.8595) (5.8936, -4.1664) knots 0 0 0 0 1 1 1 1
  spline S1002 degree 3 poles (5.8936, -4.1664) (6.0109, -4.2927) (6.1463, -4.392) (6.2005, -4.392) knots 0 0 0 0 1 1 1 1
  spline S1003 degree 3 poles (6.2005, -4.392) (6.2546, -4.392) (6.2456, -4.3469) (6.1824, -4.2837) knots 0 0 0 0 1 1 1 1
  spline S1004 degree 3 poles (6.1824, -4.2837) (6.02, -4.1212) (6.047, -3.9588) (6.2546, -3.8956) knots 0 0 0 0 1 1 1 1
  spline S1005 degree 3 poles (6.2546, -3.8956) (6.3539, -3.8595) (6.4171, -3.8054) (6.39, -3.7602) knots 0 0 0 0 1 1 1 1
  spline S1006 degree 3 poles (6.39, -3.7602) (6.3629, -3.7151) (6.2275, -3.7241) (6.0831, -3.7693) knots 0 0 0 0 1 1 1 1
  spline S1007 degree 3 poles (6.0831, -3.7693) (5.686, -3.9046) (5.1716, -3.67) (5.1716, -3.3451) knots 0 0 0 0 1 1 1 1
  line L68 (5.1716, -3.3451) -> (5.1716, -3.1014)
  line L69 (5.1716, -3.1014) -> (6.3629, -3.1465)
  spline S1008 degree 3 poles (6.3629, -3.1465) (7.852, -3.2097) (8.0235, -3.2729) (8.186, -3.8866) knots 0 0 0 0 1 1 1 1
  spline S1009 degree 3 poles (8.186, -3.8866) (8.4477, -4.8523) (8.4387, -5.1411) (8.1499, -4.7981) knots 0 0 0 0 1 1 1 1
  spline S1010 degree 3 poles (8.1499, -4.7981) (8.0867, -4.7169) (7.9784, -4.6718) (7.9152, -4.6988) knots 0 0 0 0 1 1 1 1
  spline S1011 degree 3 poles (7.9152, -4.6988) (7.843, -4.7259) (7.7167, -4.5996) (7.5993, -4.392) knots 0 0 0 0 1 1 1 1
  spline S1012 degree 3 poles (7.5993, -4.392) (7.482, -4.1934) (7.3647, -4.031) (7.3286, -4.031) knots 0 0 0 0 1 1 1 1
  spline S1013 degree 3 poles (7.3286, -4.031) (7.3015, -4.031) (7.2203, -4.2115) (7.1571, -4.4371) knots 0 0 0 0 1 1 1 1
  spline S1014 degree 3 poles (7.1571, -4.4371) (7.0398, -4.8432) (6.9225, -4.9335) (6.7329, -4.744) knots 0 0 0 0 1 1 1 1
  spline S1015 degree 3 poles (6.7329, -4.744) (6.6607, -4.6718) (6.6066, -4.6988) (6.5254, -4.8523) knots 0 0 0 0 1 1 1 1
  spline S1016 degree 3 poles (6.5254, -4.8523) (6.4622, -4.9696) (6.399, -5.0869) (6.381, -5.105) knots 0 0 0 0 1 1 1 1
  spline S1017 degree 3 poles (6.381, -5.105) (6.3719, -5.123) (6.2366, -5.0508) (6.0922, -4.9425) knots 0 0 0 0 1 1 1 1
  spline S1018 degree 3 poles (6.0922, -4.9425) (5.7943, -4.7349) (5.7131, -4.771) (5.7131, -5.0959) knots 0 0 0 0 1 1 1 1
  spline S1019 degree 3 poles (5.7131, -5.0959) (5.7131, -5.2674) (5.677, -5.3035) (5.5326, -5.2674) knots 0 0 0 0 1 1 1 1
  spline S1020 degree 3 poles (5.5326, -5.2674) (5.4153, -5.2403) (5.316, -5.2945) (5.2167, -5.4389) knots 0 0 0 0 1 1 1 1
  spline S1021 degree 3 poles (5.2167, -5.4389) (5.1175, -5.6013) (4.9911, -5.6555) (4.7655, -5.6555) knots 0 0 0 0 1 1 1 1
  spline S1022 degree 3 poles (4.7655, -5.6555) (4.603, -5.6555) (4.4045, -5.7096) (4.3413, -5.7728) knots 0 0 0 0 1 1 1 1
  spline S1023 degree 3 poles (4.3413, -5.7728) (3.881, -6.206) (3.4298, -6.3053) (3.0959, -6.0345) knots 0 0 0 0 1 1 1 1
  spline S1024 degree 3 poles (7.3557, -6.4046) (7.3015, -6.3865) (7.1932, -6.3865) (7.13, -6.4046) knots 0 0 0 0 1 1 1 1
  spline S1025 degree 3 poles (7.13, -6.4046) (7.0759, -6.4316) (7.121, -6.4497) (7.2474, -6.4497) knots 0 0 0 0 1 1 1 1
  spline S1026 degree 3 poles (7.2474, -6.4497) (7.3737, -6.4497) (7.4188, -6.4316) (7.3557, -6.4046) knots 0 0 0 0 1 1 1 1
  spline S1027 degree 3 poles (16.5882, -5.1411) (16.6243, -4.9967) (16.7056, -4.7801) (16.7778, -4.6447) knots 0 0 0 0 1 1 1 1
  spline S1028 degree 3 poles (16.7778, -4.6447) (16.85, -4.5183) (16.9041, -4.3378) (16.9041, -4.2386) knots 0 0 0 0 1 1 1 1
  spline S1029 degree 3 poles (16.9041, -4.2386) (16.8951, -4.0851) (16.8951, -4.0851) (16.8048, -4.2386) knots 0 0 0 0 1 1 1 1
  spline S1030 degree 3 poles (16.8048, -4.2386) (16.7597, -4.3198) (16.6604, -4.392) (16.5882, -4.392) knots 0 0 0 0 1 1 1 1
  spline S1031 degree 3 poles (16.5882, -4.392) (16.3987, -4.392) (16.3536, -4.5274) (16.4529, -4.7891) knots 0 0 0 0 1 1 1 1
  spline S1032 degree 3 poles (16.4529, -4.7891) (16.507, -4.9335) (16.507, -5.0328) (16.4529, -5.0689) knots 0 0 0 0 1 1 1 1
  spline S1033 degree 3 poles (16.4529, -5.0689) (16.3355, -5.1411) (16.3355, -5.3847) (16.4529, -5.3847) knots 0 0 0 0 1 1 1 1
  spline S1034 degree 3 poles (16.4529, -5.3847) (16.498, -5.3847) (16.5612, -5.2764) (16.5882, -5.1411) knots 0 0 0 0 1 1 1 1
  spline S1035 degree 3 poles (17.3102, -3.7602) (17.2832, -3.7151) (17.238, -3.67) (17.211, -3.67) knots 0 0 0 0 1 1 1 1
  spline S1036 degree 3 poles (17.211, -3.67) (17.1929, -3.67) (17.1749, -3.7151) (17.1749, -3.7602) knots 0 0 0 0 1 1 1 1
  spline S1037 degree 3 poles (17.1749, -3.7602) (17.1749, -3.8144) (17.22, -3.8505) (17.2741, -3.8505) knots 0 0 0 0 1 1 1 1
  spline S1038 degree 3 poles (17.2741, -3.8505) (17.3193, -3.8505) (17.3373, -3.8144) (17.3102, -3.7602) knots 0 0 0 0 1 1 1 1
  spline S1039 degree 3 poles (18.1044, -3.318) (18.4203, -3.1285) (18.5015, -3.0473) (18.4023, -3.0112) knots 0 0 0 0 1 1 1 1
  spline S1040 degree 3 poles (18.4023, -3.0112) (18.2218, -2.939) (18.2127, -2.6863) (18.3932, -2.6231) knots 0 0 0 0 1 1 1 1
  spline S1041 degree 3 poles (18.3932, -2.6231) (18.5737, -2.5509) (18.4023, -2.3162) (18.1766, -2.3162) knots 0 0 0 0 1 1 1 1
  spline S1042 degree 3 poles (18.1766, -2.3162) (17.9781, -2.3162) (17.6081, -2.578) (17.6712, -2.6772) knots 0 0 0 0 1 1 1 1
  spline S1043 degree 3 poles (17.6712, -2.6772) (17.6983, -2.7133) (17.6442, -2.7314) (17.5449, -2.7043) knots 0 0 0 0 1 1 1 1
  spline S1044 degree 3 poles (17.5449, -2.7043) (17.3012, -2.6411) (17.229, -2.8216) (17.4456, -2.9751) knots 0 0 0 0 1 1 1 1
  spline S1045 degree 3 poles (17.4456, -2.9751) (17.59, -3.0743) (17.6171, -3.1646) (17.572, -3.3451) knots 0 0 0 0 1 1 1 1
  spline S1046 degree 3 poles (17.572, -3.3451) (17.4998, -3.6339) (17.5629, -3.6339) (18.1044, -3.318) knots 0 0 0 0 1 1 1 1
  spline S1047 degree 3 poles (-16.714, -3.1285) (-16.6869, -3.0834) (-16.7411, -3.0382) (-16.8404, -3.0382) knots 0 0 0 0 1 1 1 1
  spline S1048 degree 3 poles (-16.8404, -3.0382) (-16.9487, -3.0382) (-17.0299, -3.0834) (-17.0299, -3.1285) knots 0 0 0 0 1 1 1 1
  spline S1049 degree 3 poles (-17.0299, -3.1285) (-17.0299, -3.1826) (-16.9757, -3.2187) (-16.9035, -3.2187) knots 0 0 0 0 1 1 1 1
  spline S1050 degree 3 poles (-16.9035, -3.2187) (-16.8313, -3.2187) (-16.7411, -3.1826) (-16.714, -3.1285) knots 0 0 0 0 1 1 1 1
  spline S1051 degree 3 poles (-12.2466, -3.0292) (-12.2466, -2.9119) (-12.5896, -2.6772) (-12.752, -2.6863) knots 0 0 0 0 1 1 1 1
  spline S1052 degree 3 poles (-12.752, -2.6863) (-12.9145, -2.6863) (-12.9145, -2.6953) (-12.743, -2.7675) knots 0 0 0 0 1 1 1 1
  spline S1053 degree 3 poles (-12.743, -2.7675) (-12.5986, -2.8307) (-12.6257, -2.8487) (-12.9055, -2.8487) knots 0 0 0 0 1 1 1 1
  spline S1054 degree 3 poles (-12.9055, -2.8487) (-13.2845, -2.8577) (-13.3657, -3.0292) (-12.9957, -3.0563) knots 0 0 0 0 1 1 1 1
  spline S1055 degree 3 poles (-12.9957, -3.0563) (-12.3549, -3.0924) (-12.2466, -3.0834) (-12.2466, -3.0292) knots 0 0 0 0 1 1 1 1
  spline S1056 degree 3 poles (19.3138, -2.8397) (19.4311, -2.7855) (19.5214, -2.7043) (19.5214, -2.6502) knots 0 0 0 0 1 1 1 1
  spline S1057 degree 3 poles (19.5214, -2.6502) (19.5214, -2.5148) (18.7091, -2.6411) (18.5467, -2.8036) knots 0 0 0 0 1 1 1 1
  spline S1058 degree 3 poles (18.5467, -2.8036) (18.4113, -2.939) (18.4293, -2.948) (18.7542, -2.939) knots 0 0 0 0 1 1 1 1
  spline S1059 degree 3 poles (18.7542, -2.939) (18.9528, -2.939) (19.2055, -2.8938) (19.3138, -2.8397) knots 0 0 0 0 1 1 1 1
  spline S1060 degree 3 poles (-2.5989, -2.6863) (-2.5267, -2.6411) (-2.5177, -2.587) (-2.5718, -2.5509) knots 0 0 0 0 1 1 1 1
  spline S1061 degree 3 poles (-2.5718, -2.5509) (-2.6982, -2.4787) (-2.9599, -2.587) (-2.8967, -2.6863) knots 0 0 0 0 1 1 1 1
  spline S1062 degree 3 poles (-2.8967, -2.6863) (-2.8336, -2.7855) (-2.7614, -2.7855) (-2.5989, -2.6863) knots 0 0 0 0 1 1 1 1
  spline S1063 degree 3 poles (17.1207, -2.5599) (17.0936, -2.4697) (17.0395, -2.4245) (17.0124, -2.4516) knots 0 0 0 0 1 1 1 1
  spline S1064 degree 3 poles (17.0124, -2.4516) (16.9853, -2.4787) (17.0124, -2.5509) (17.0756, -2.6141) knots 0 0 0 0 1 1 1 1
  spline S1065 degree 3 poles (17.0756, -2.6141) (17.1658, -2.6953) (17.1749, -2.6863) (17.1207, -2.5599) knots 0 0 0 0 1 1 1 1
  spline S1066 degree 3 poles (-3.1133, -2.6141) (-3.1765, -2.587) (-3.2577, -2.596) (-3.2848, -2.6231) knots 0 0 0 0 1 1 1 1
  spline S1067 degree 3 poles (-3.2848, -2.6231) (-3.3209, -2.6502) (-3.2668, -2.6772) (-3.1675, -2.6682) knots 0 0 0 0 1 1 1 1
  spline S1068 degree 3 poles (-3.1675, -2.6682) (-3.0682, -2.6682) (-3.0411, -2.6411) (-3.1133, -2.6141) knots 0 0 0 0 1 1 1 1
  spline S1069 degree 3 poles (-15.0444, -2.587) (-15.0444, -2.5419) (-15.0805, -2.4967) (-15.1256, -2.4967) knots 0 0 0 0 1 1 1 1
  spline S1070 degree 3 poles (-15.1256, -2.4967) (-15.1798, -2.4967) (-15.2429, -2.5419) (-15.27, -2.587) knots 0 0 0 0 1 1 1 1
  spline S1071 degree 3 poles (-15.27, -2.587) (-15.2971, -2.6411) (-15.261, -2.6772) (-15.1888, -2.6772) knots 0 0 0 0 1 1 1 1
  spline S1072 degree 3 poles (-15.1888, -2.6772) (-15.1076, -2.6772) (-15.0444, -2.6411) (-15.0444, -2.587) knots 0 0 0 0 1 1 1 1
  spline S1073 degree 3 poles (1.706, -2.2711) (1.697, -1.9372) (1.5345, -1.8108) (1.2548, -1.9191) knots 0 0 0 0 1 1 1 1
  spline S1074 degree 3 poles (1.2548, -1.9191) (1.0382, -2.0004) (1.0743, -2.1718) (1.3811, -2.3884) knots 0 0 0 0 1 1 1 1
  spline S1075 degree 3 poles (1.3811, -2.3884) (1.5255, -2.4967) (1.6609, -2.587) (1.6789, -2.587) knots 0 0 0 0 1 1 1 1
  spline S1076 degree 3 poles (1.6789, -2.587) (1.697, -2.587) (1.706, -2.4426) (1.706, -2.2711) knots 0 0 0 0 1 1 1 1
  spline S1077 degree 3 poles (21.4346, -2.2711) (21.6151, -2.1448) (21.8137, -2.0455) (21.8678, -2.0455) knots 0 0 0 0 1 1 1 1
  spline S1078 degree 3 poles (21.8678, -2.0455) (21.9852, -2.0455) (22.4093, -1.6033) (22.4093, -1.4859) knots 0 0 0 0 1 1 1 1
  spline S1079 degree 3 poles (22.4093, -1.4859) (22.4093, -1.3867) (21.94, -1.6935) (21.57, -2.0365) knots 0 0 0 0 1 1 1 1
  spline S1080 degree 3 poles (21.57, -2.0365) (21.4346, -2.1628) (21.209, -2.3162) (21.0736, -2.3704) knots 0 0 0 0 1 1 1 1
  spline S1081 degree 3 poles (21.0736, -2.3704) (20.9383, -2.4336) (20.8931, -2.4877) (20.9653, -2.4877) knots 0 0 0 0 1 1 1 1
  spline S1082 degree 3 poles (20.9653, -2.4877) (21.0466, -2.4967) (21.2541, -2.3975) (21.4346, -2.2711) knots 0 0 0 0 1 1 1 1
  spline S1083 degree 3 poles (20.108, -2.4065) (20.1351, -2.3614) (20.126, -2.3162) (20.0719, -2.3162) knots 0 0 0 0 1 1 1 1
  spline S1084 degree 3 poles (20.0719, -2.3162) (20.0268, -2.3162) (19.9546, -2.3614) (19.9275, -2.4065) knots 0 0 0 0 1 1 1 1
  spline S1085 degree 3 poles (19.9275, -2.4065) (19.9004, -2.4606) (19.9094, -2.4967) (19.9636, -2.4967) knots 0 0 0 0 1 1 1 1
  spline S1086 degree 3 poles (19.9636, -2.4967) (20.0087, -2.4967) (20.0809, -2.4606) (20.108, -2.4065) knots 0 0 0 0 1 1 1 1
  spline S1087 degree 3 poles (0.0274, -2.4065) (0.1447, -2.3343) (0.1447, -2.3162) (0.0093, -2.3162) knots 0 0 0 0 1 1 1 1
  spline S1088 degree 3 poles (0.0093, -2.3162) (-0.0719, -2.3162) (-0.1712, -2.3614) (-0.1983, -2.4065) knots 0 0 0 0 1 1 1 1
  spline S1089 degree 3 poles (-0.1983, -2.4065) (-0.2705, -2.5238) (-0.1531, -2.5238) (0.0274, -2.4065) knots 0 0 0 0 1 1 1 1
  spline S1090 degree 3 poles (-1.1008, -2.4065) (-1.0737, -2.3614) (-0.9293, -2.3162) (-0.7849, -2.3162) knots 0 0 0 0 1 1 1 1
  spline S1091 degree 3 poles (-0.7849, -2.3162) (-0.6224, -2.3162) (-0.3156, -2.1718) (0.0274, -1.9372) knots 0 0 0 0 1 1 1 1
  spline S1092 degree 3 poles (0.0274, -1.9372) (0.3252, -1.7206) (0.6681, -1.495) (0.7764, -1.4408) knots 0 0 0 0 1 1 1 1
  spline S1093 degree 3 poles (0.7764, -1.4408) (1.0652, -1.2784) (0.7584, -1.2964) (0.4425, -1.4589) knots 0 0 0 0 1 1 1 1
  spline S1094 degree 3 poles (0.4425, -1.4589) (0.3071, -1.5311) (0.0364, -1.5942) (-0.1531, -1.5942) knots 0 0 0 0 1 1 1 1
  spline S1095 degree 3 poles (-0.1531, -1.5942) (-0.4149, -1.5942) (-0.5502, -1.6484) (-0.7127, -1.8469) knots 0 0 0 0 1 1 1 1
  spline S1096 degree 3 poles (-0.7127, -1.8469) (-0.821, -1.9823) (-1.0647, -2.1538) (-1.2361, -2.217) knots 0 0 0 0 1 1 1 1
  spline S1097 degree 3 poles (-1.2361, -2.217) (-1.6964, -2.3975) (-1.7686, -2.4967) (-1.4437, -2.4967) knots 0 0 0 0 1 1 1 1
  spline S1098 degree 3 poles (-1.4437, -2.4967) (-1.2813, -2.4967) (-1.1278, -2.4606) (-1.1008, -2.4065) knots 0 0 0 0 1 1 1 1
  spline S1099 degree 3 poles (-13.9614, -2.3162) (-13.3748, -2.1177) (-12.6076, -1.7025) (-12.6076, -1.5852) knots 0 0 0 0 1 1 1 1
  spline S1100 degree 3 poles (-12.6076, -1.5852) (-12.6076, -1.4589) (-12.9055, -1.495) (-13.095, -1.6394) knots 0 0 0 0 1 1 1 1
  spline S1101 degree 3 poles (-13.095, -1.6394) (-13.1943, -1.7116) (-13.3387, -1.7747) (-13.4109, -1.7747) knots 0 0 0 0 1 1 1 1
  spline S1102 degree 3 poles (-13.4109, -1.7747) (-13.5101, -1.7657) (-13.4921, -1.7386) (-13.3567, -1.6574) knots 0 0 0 0 1 1 1 1
  spline S1103 degree 3 poles (-13.3567, -1.6574) (-13.2304, -1.5852) (-13.1852, -1.504) (-13.2304, -1.4318) knots 0 0 0 0 1 1 1 1
  spline S1104 degree 3 poles (-13.2304, -1.4318) (-13.2845, -1.3415) (-13.3296, -1.3596) (-13.4379, -1.4769) knots 0 0 0 0 1 1 1 1
  spline S1105 degree 3 poles (-13.4379, -1.4769) (-13.5101, -1.5672) (-13.6004, -1.7116) (-13.6275, -1.8018) knots 0 0 0 0 1 1 1 1
  spline S1106 degree 3 poles (-13.6275, -1.8018) (-13.6636, -1.883) (-13.7628, -1.9552) (-13.8621, -1.9552) knots 0 0 0 0 1 1 1 1
  spline S1107 degree 3 poles (-13.8621, -1.9552) (-13.9614, -1.9552) (-14.0697, -2.0004) (-14.1058, -2.0545) knots 0 0 0 0 1 1 1 1
  spline S1108 degree 3 poles (-14.1058, -2.0545) (-14.1329, -2.1087) (-14.2863, -2.226) (-14.4487, -2.3253) knots 0 0 0 0 1 1 1 1
  spline S1109 degree 3 poles (-14.4487, -2.3253) (-14.8007, -2.5419) (-14.6022, -2.5419) (-13.9614, -2.3162) knots 0 0 0 0 1 1 1 1
  line L70 (20.6946, -2.226) -> (20.9202, -2.0455)
  line L71 (20.9202, -2.0455) -> (20.5682, -2.0455)
  spline S1110 degree 3 poles (20.5682, -2.0455) (20.2524, -2.0455) (20.2343, -2.0635) (20.3426, -2.2079) knots 0 0 0 0 1 1 1 1
  spline S1111 degree 3 poles (20.3426, -2.2079) (20.4058, -2.2892) (20.469, -2.3704) (20.469, -2.3794) knots 0 0 0 0 1 1 1 1
  spline S1112 degree 3 poles (20.469, -2.3794) (20.469, -2.3884) (20.5682, -2.3162) (20.6946, -2.226) knots 0 0 0 0 1 1 1 1
  spline S1113 degree 3 poles (19.8824, -2.226) (19.9907, -2.1538) (19.9816, -2.1357) (19.8192, -2.1357) knots 0 0 0 0 1 1 1 1
  spline S1114 degree 3 poles (19.8192, -2.1357) (19.7109, -2.1357) (19.5936, -2.1809) (19.5665, -2.226) knots 0 0 0 0 1 1 1 1
  spline S1115 degree 3 poles (19.5665, -2.226) (19.4943, -2.3433) (19.7019, -2.3433) (19.8824, -2.226) knots 0 0 0 0 1 1 1 1
  spline S1116 degree 3 poles (-12.7881, -2.226) (-12.7881, -2.1809) (-12.8423, -2.1357) (-12.9145, -2.1357) knots 0 0 0 0 1 1 1 1
  spline S1117 degree 3 poles (-12.9145, -2.1357) (-12.9867, -2.1357) (-13.0769, -2.1809) (-13.104, -2.226) knots 0 0 0 0 1 1 1 1
  spline S1118 degree 3 poles (-13.104, -2.226) (-13.1311, -2.2801) (-13.0769, -2.3162) (-12.9777, -2.3162) knots 0 0 0 0 1 1 1 1
  spline S1119 degree 3 poles (-12.9777, -2.3162) (-12.8694, -2.3162) (-12.7881, -2.2801) (-12.7881, -2.226) knots 0 0 0 0 1 1 1 1
  spline S1120 degree 3 poles (22.5267, -2.0996) (22.6079, -2.0365) (22.7794, -2.0004) (22.8877, -2.0184) knots 0 0 0 0 1 1 1 1
  spline S1121 degree 3 poles (22.8877, -2.0184) (23.023, -2.0455) (23.2757, -1.9552) (23.5645, -1.7747) knots 0 0 0 0 1 1 1 1
  spline S1122 degree 3 poles (23.5645, -1.7747) (23.8172, -1.6213) (24.0699, -1.513) (24.1151, -1.5401) knots 0 0 0 0 1 1 1 1
  spline S1123 degree 3 poles (24.1151, -1.5401) (24.2143, -1.6033) (24.4219, -1.3596) (24.44, -1.152) knots 0 0 0 0 1 1 1 1
  spline S1124 degree 3 poles (24.44, -1.152) (24.449, -1.0166) (24.3317, -1.0708) (23.8624, -1.3776) knots 0 0 0 0 1 1 1 1
  spline S1125 degree 3 poles (23.8624, -1.3776) (23.4382, -1.6664) (23.1855, -1.7747) (22.9508, -1.7747) knots 0 0 0 0 1 1 1 1
  spline S1126 degree 3 poles (22.9508, -1.7747) (22.7342, -1.7747) (22.5628, -1.8379) (22.4545, -1.9552) knots 0 0 0 0 1 1 1 1
  spline S1127 degree 3 poles (22.4545, -1.9552) (22.2559, -2.1718) (22.301, -2.2621) (22.5267, -2.0996) knots 0 0 0 0 1 1 1 1
  spline S1128 degree 3 poles (-2.9058, -2.0365) (-2.7072, -1.9913) (-2.3462, -1.9372) (-2.1116, -1.9101) knots 0 0 0 0 1 1 1 1
  spline S1129 degree 3 poles (-2.1116, -1.9101) (-1.8228, -1.874) (-1.5881, -1.7657) (-1.3896, -1.6033) knots 0 0 0 0 1 1 1 1
  spline S1130 degree 3 poles (-1.3896, -1.6033) (-1.2271, -1.4589) (-0.9564, -1.3235) (-0.7759, -1.2874) knots 0 0 0 0 1 1 1 1
  spline S1131 degree 3 poles (-0.7759, -1.2874) (-0.5954, -1.2603) (-0.3788, -1.152) (-0.2885, -1.0527) knots 0 0 0 0 1 1 1 1
  spline S1132 degree 3 poles (-0.2885, -1.0527) (-0.1983, -0.9535) (-0.0539, -0.8722) (0.0364, -0.8722) knots 0 0 0 0 1 1 1 1
  spline S1133 degree 3 poles (0.0364, -0.8722) (0.2079, -0.8722) (1.0201, -0.5473) (1.0201, -0.4751) knots 0 0 0 0 1 1 1 1
  spline S1134 degree 3 poles (1.0201, -0.4751) (1.0201, -0.4481) (0.9118, -0.4661) (0.7674, -0.5112) knots 0 0 0 0 1 1 1 1
  spline S1135 degree 3 poles (0.7674, -0.5112) (0.632, -0.5473) (0.253, -0.6105) (-0.0809, -0.6376) knots 0 0 0 0 1 1 1 1
  spline S1136 degree 3 poles (-0.0809, -0.6376) (-0.7127, -0.7008) (-1.7596, -1.152) (-2.0574, -1.504) knots 0 0 0 0 1 1 1 1
  spline S1137 degree 3 poles (-2.0574, -1.504) (-2.2199, -1.6935) (-3.1133, -1.874) (-3.005, -1.6935) knots 0 0 0 0 1 1 1 1
  spline S1138 degree 3 poles (-3.005, -1.6935) (-2.8697, -1.4859) (-3.2216, -1.6033) (-3.4924, -1.865) knots 0 0 0 0 1 1 1 1
  line L72 (-3.4924, -1.865) -> (-3.7722, -2.1357)
  line L73 (-3.7722, -2.1357) -> (-3.5195, -2.1267)
  spline S1139 degree 3 poles (-3.5195, -2.1267) (-3.3841, -2.1177) (-3.1043, -2.0816) (-2.9058, -2.0365) knots 0 0 0 0 1 1 1 1
  spline S1140 degree 3 poles (-15.1437, -2.0545) (-15.0354, -1.9823) (-15.0624, -1.9552) (-15.252, -1.9011) knots 0 0 0 0 1 1 1 1
  spline S1141 degree 3 poles (-15.252, -1.9011) (-15.5227, -1.8379) (-15.64, -1.8921) (-15.5408, -2.0365) knots 0 0 0 0 1 1 1 1
  spline S1142 degree 3 poles (-15.5408, -2.0365) (-15.4686, -2.1538) (-15.3151, -2.1628) (-15.1437, -2.0545) knots 0 0 0 0 1 1 1 1
  spline S1143 degree 3 poles (19.4492, -1.9823) (19.386, -1.9552) (19.3048, -1.9643) (19.2777, -1.9913) knots 0 0 0 0 1 1 1 1
  spline S1144 degree 3 poles (19.2777, -1.9913) (19.2416, -2.0184) (19.2957, -2.0455) (19.395, -2.0365) knots 0 0 0 0 1 1 1 1
  spline S1145 degree 3 poles (19.395, -2.0365) (19.4943, -2.0365) (19.5214, -2.0094) (19.4492, -1.9823) knots 0 0 0 0 1 1 1 1
  spline S1146 degree 3 poles (6.9495, -1.7747) (6.9134, -1.6484) (6.8864, -1.4137) (6.8864, -1.2513) knots 0 0 0 0 1 1 1 1
  spline S1147 degree 3 poles (6.8864, -1.2513) (6.8864, -1.0257) (6.8322, -0.9354) (6.6517, -0.8542) knots 0 0 0 0 1 1 1 1
  spline S1148 degree 3 poles (6.6517, -0.8542) (6.5254, -0.791) (6.3629, -0.6466) (6.2997, -0.5203) knots 0 0 0 0 1 1 1 1
  spline S1149 degree 3 poles (6.2997, -0.5203) (6.1824, -0.3037) (6.1734, -0.3037) (6.1644, -0.4751) knots 0 0 0 0 1 1 1 1
  spline S1150 degree 3 poles (6.1644, -0.4751) (6.1644, -0.5834) (6.2817, -0.8361) (6.4351, -1.0347) knots 0 0 0 0 1 1 1 1
  spline S1151 degree 3 poles (6.4351, -1.0347) (6.5795, -1.2423) (6.7059, -1.4859) (6.7059, -1.5852) knots 0 0 0 0 1 1 1 1
  spline S1152 degree 3 poles (6.7059, -1.5852) (6.7059, -1.6755) (6.7781, -1.8108) (6.8593, -1.874) knots 0 0 0 0 1 1 1 1
  spline S1153 degree 3 poles (6.8593, -1.874) (6.9947, -1.9913) (7.0037, -1.9733) (6.9495, -1.7747) knots 0 0 0 0 1 1 1 1
  spline S1154 degree 3 poles (5.0814, -1.6845) (5.0814, -1.5401) (4.4135, -0.8722) (4.2781, -0.8722) knots 0 0 0 0 1 1 1 1
  spline S1155 degree 3 poles (4.2781, -0.8722) (4.0886, -0.8722) (4.1789, -1.0437) (4.4225, -1.161) knots 0 0 0 0 1 1 1 1
  spline S1156 degree 3 poles (4.4225, -1.161) (4.5579, -1.2242) (4.6933, -1.3776) (4.7204, -1.504) knots 0 0 0 0 1 1 1 1
  spline S1157 degree 3 poles (4.7204, -1.504) (4.7745, -1.7296) (5.0814, -1.883) (5.0814, -1.6845) knots 0 0 0 0 1 1 1 1
  spline S1158 degree 3 poles (4.3323, -1.5311) (4.5218, -1.4589) (4.4677, -1.3506) (4.1337, -1.152) knots 0 0 0 0 1 1 1 1